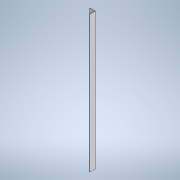
# Autodesk Inventor part: Stanik1000
Saved by Autodesk Inventor 2020.1 (Build 241239000, 239)
## iProperties
Created: 2023-01-06
Part Number: Stanik1000
Material: Типовые
Document SubType Name: Modeling
Designer: KirikDK
Density: 1 g/cm^3
Appearance: По умолчанию
Author: KirikDK
Autodesk Inventor part; units mm, degrees
ref_plane "YZ Plane" through (0, 0, 0) normal (1, 0, 0) x (0, 1, 0)
ref_plane "XZ Plane" through (0, 0, 0) normal (0, 1, 0) x (-1, 0, 0)
ref_plane "XY Plane" through (0, 0, 0) normal (0, 0, 1) x (1, 0, 0)
sketch "Эскиз1" plane through (0, 0, 0) normal (0, 1, 0) x (-1, 0, 0)
  line L0 (0, 40) -> (0, 0)
  line L1 (0, 0) -> (40, 0)
  line L2 (40, 0) -> (40, 3)
  line L3 (40, 3) -> (3, 3)
  line L4 (3, 3) -> (3, 40)
  line L5 (3, 40) -> (0, 40)
  dimension "d0" = 3
  dimension "d1" = 3
  dimension "d2" = 40
  dimension "d3" = 40
  constraints: 12 end point, 2 perpendicular, 2 vertical
  measures "d0" distance of L1.end L2.end
  measures "d1" distance of L4.end L0.start
  measures "d2" distance of L0.start L0.end
  measures "d3" distance of L0.end L1.end
extrude "Выдавливание1" add sketch "Эскиз1" along normal blind 1000
